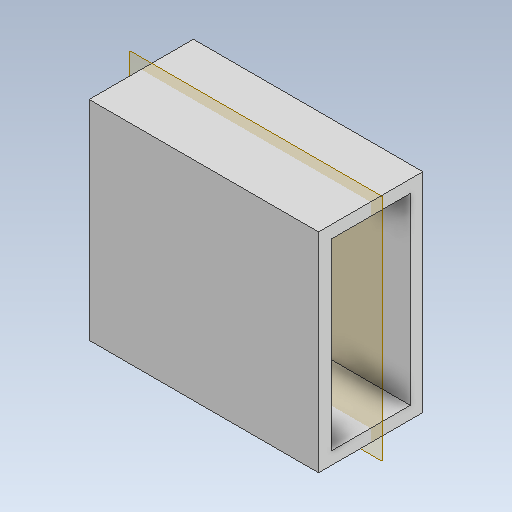
# Autodesk Inventor part: SIDEBUMPERMOUNTING
Saved by Autodesk Inventor 2020 (Build 240168000, 168)
## iProperties
Created: 2021-01-20
Part Number: SIDEBUMPERMOUNTING
Material: Generic
Document SubType Name: Modeling
Designer: lucky
Density: 1 g/cm^3
Appearance: Default
Mass: 22.77 g
Surface Area: 160.08 cm^2
Volume: 22.77 cm^3
Author: lucky
Autodesk Inventor part; units mm, degrees
ref_plane "YZ Plane" through (0, 0, 0) normal (1, 0, 0) x (0, 1, 0)
ref_plane "XZ Plane" through (0, 0, 0) normal (0, 1, 0) x (-1, 0, 0)
sketch "Sketch1" plane through (0, 0, 0) normal (1, 0, 0) x (0, 1, 0)
  line L0 (-25, 12.5) -> (25, 12.5)
  line L1 (25, 12.5) -> (25, -12.5)
  line L2 (25, -12.5) -> (-25, -12.5)
  line L3 (-25, -12.5) -> (-25, 12.5)
  line L4 (-25, 12.5) -> (25, -12.5) construction
  line L5 (25, 12.5) -> (-25, -12.5) construction
  line L6 (22, -9.5) -> (22, 9.5)
  line L7 (22, 9.5) -> (-22, 9.5)
  line L8 (-22, 9.5) -> (-22, -9.5)
  line L9 (-22, -9.5) -> (22, -9.5)
  point P0 (0, 0)
  dimension "d0" = 25
  dimension "d1" = 50
  dimension "d2" = 3
  constraints: 20 end point, 4 parallel, 2 midpoint, 2 perpendicular, 1 horizontal, 3 other
  measures "d0" distance between parallel lines of L2 L0
  measures "d1" distance between parallel lines of L3 L1
  measures "d2" distance between parallel lines of L1 L6
extrude "Extrusion1" add sketch "Sketch1" along normal mid plane 55
equation "\"d3\" = WheelBay_Depth"
equation "\"WheelBay_Depth\" = 55"
equation "\"Chassi_GroundClearance\" = 10.116"
equation "\"Wheel_Diametre\" = 152.4"
equation "\"Wheel_Seperation\" = 285.75"
equation "\"Wheel_HeightOffset\" = 4"
equation "\"Wheel_Clearance\" = 13.05"
equation "\"Wheel_CentreDrop\" = 4"
equation "\"Wheel_Diametre2\" = 101.6"
equation "\"Wheel_Seperation2\" = 194.33333"
equation "\"Wheel_HeightOffset2\" = 4"
equation "\"Wheel_Clearance2\" = 32.7"
equation "\"Chain_Pitch\" = 9.525"
equation "\"Wheel_CCSpan\" = 571.5"
equation "\"Wheel_CCSpan2\" = 471.5"
equation "\"Wheel_MaxSeperation\" = 285.75"
equation "\"Wheel_MaxSeperation2\" = 190.5"
equation "\"MotorholeCC\" = 95.25"
equation "\"Heightfromcenter\" = 6.7125"
equation "\"MotorholeHorizontal\" = 95.01318"
equation "\"OutputshaftTopOffset\" = 30.058"
equation "\"Chassi_SideRivetSpacing\" = 37.5"
equation "\"Sprocket_Thickness\" = 10.668"
equation "\"BumperMountingBarOffset\" = 177.8"
body "Solid1"
